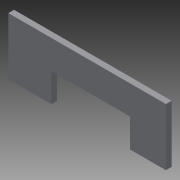
# Autodesk Inventor part: Different Sweep
Saved by Autodesk Inventor 2014 (Build 180170000, 170)
## iProperties
Created: 2014-03-20
Part Number: Different Sweep
Material: Generic
Document SubType Name: Modeling
Designer: Pranav
Density: 1 g/cm^3
Appearance: Default
Author: Pranav
Autodesk Inventor part; units mm, degrees
ref_plane "YZ Plane" through (0, 0, 0) normal (1, 0, 0) x (0, 1, 0)
ref_plane "XZ Plane" through (0, 0, 0) normal (0, 1, 0) x (-1, 0, 0)
ref_plane "XY Plane" through (0, 0, 0) normal (0, 0, 1) x (1, 0, 0)
sketch "Sketch3" plane through (0, 0, 0) normal (0, 0, 1) x (1, 0, 0)
  line L0 (0, 0) -> (0, 25.4)
  line L1 (0, 0) -> (19.05, 0)
  line L2 (0, 25.4) -> (69.85, 25.4)
  line L3 (69.85, 25.4) -> (69.85, 0)
  line L4 (69.85, 0) -> (53.975, 0)
  line L5 (53.975, 0) -> (53.975, 12.7)
  line L6 (53.975, 12.7) -> (19.05, 12.7)
  line L7 (19.05, 12.7) -> (19.05, 0)
  dimension "d7" = 25.4
  dimension "d8" = 69.85
  constraints: 16 end point, 4 parallel, 2 perpendicular, 1 vertical
  measures "d7" distance of L0.start L0.end
  measures "d8" distance of L0.end L2.end
extrude "Extrusion2" add sketch "Sketch3" along normal blind 2.54
body "Solid2"
